Autodesk Inventor part; units mm, degrees
(part 2 of 3)
sketch "Sketch14" plane through (-2.25, 0, -155) normal (0, 0, -1) x (-1, 0, 0)
  line L0 (27.5213, 34.6376) -> (93.9787, 34.6376) construction
  line L1 (93.9787, 34.6376) -> (93.9787, 30.375) construction
  line L2 (93.9787, 30.375) -> (27.5213, 30.375) construction
  line L3 (27.5213, 30.375) -> (27.5213, 34.6376) construction
  line L4 (107.75, 0) -> (107.75, 55) projected
  circle A0 centre (60.75, 23) radius 5.375 projected
  spline S0 degree 2 poles (33.5458, 31.2786) (33.5458, 30.8312) (33.2054, 30.1457) (32.9234, 29.922) knots 0 0 0 1 2 2 2
  spline S1 degree 2 poles (32.9234, 29.922) (32.5831, 29.6594) (31.81, 29.4358) (31.1973, 29.4358) knots 0 0 0 1 2 2 2
  line L5 (31.1973, 29.4358) -> (29.4761, 29.4358)
  line L6 (29.4761, 29.4358) -> (29.4761, 35.4358)
  line L7 (29.4761, 35.4358) -> (31.066, 35.4358)
  spline S2 degree 2 poles (31.066, 35.4358) (31.7079, 35.4358) (32.3497, 35.3531) (32.6414, 35.1927) knots 0 0 0 1 2 2 2
  spline S3 degree 2 poles (32.6414, 35.1927) (32.9672, 35.0225) (33.2638, 34.4633) (33.2638, 34.0841) knots 0 0 0 1 2 2 2
  spline S4 degree 2 poles (33.2638, 34.0841) (33.2638, 33.6611) (32.8164, 32.9901) (32.4226, 32.8004) knots 0 0 0 1 2 2 2
  line L8 (32.4226, 32.8004) -> (32.4226, 32.7713)
  spline S5 degree 2 poles (32.4226, 32.7713) (32.9575, 32.6254) (33.5458, 31.8523) (33.5458, 31.2786) knots 0 0 0 1 2 2 2
  spline S6 degree 2 poles (32.7143, 31.2445) (32.7143, 31.5849) (32.5199, 32.0225) (32.2281, 32.1781) knots 0 0 0 1 2 2 2
  spline S7 degree 2 poles (32.2281, 32.1781) (32.0385, 32.2753) (31.5912, 32.3337) (31.1779, 32.3337) knots 0 0 0 1 2 2 2
  line L9 (31.1779, 32.3337) -> (30.2735, 32.3337)
  line L10 (30.2735, 32.3337) -> (30.2735, 30.1165)
  line L11 (30.2735, 30.1165) -> (30.9202, 30.1165)
  spline S8 degree 2 poles (30.9202, 30.1165) (31.4453, 30.1165) (32.0482, 30.2137) (32.2816, 30.3693) knots 0 0 0 1 2 2 2
  spline S9 degree 2 poles (32.2816, 30.3693) (32.5053, 30.5298) (32.7143, 30.9285) (32.7143, 31.2445) knots 0 0 0 1 2 2 2
  spline S10 degree 2 poles (32.4323, 33.9722) (32.4323, 34.1862) (32.2865, 34.5071) (32.126, 34.5995) knots 0 0 0 1 2 2 2
  spline S11 degree 2 poles (32.126, 34.5995) (31.9315, 34.7064) (31.4599, 34.7551) (31.0369, 34.7551) knots 0 0 0 1 2 2 2
  line L12 (31.0369, 34.7551) -> (30.2735, 34.7551)
  line L13 (30.2735, 34.7551) -> (30.2735, 32.9998)
  line L14 (30.2735, 32.9998) -> (31.1779, 32.9998)
  spline S12 degree 2 poles (31.1779, 32.9998) (31.5523, 32.9998) (31.9072, 33.0776) (32.0968, 33.1991) knots 0 0 0 1 2 2 2
  spline S13 degree 2 poles (32.0968, 33.1991) (32.2816, 33.3158) (32.4323, 33.6902) (32.4323, 33.9722) knots 0 0 0 1 2 2 2
  spline S14 degree 2 poles (36.7889, 29.9123) (36.6965, 29.8442) (36.3853, 29.6011) (36.2395, 29.5282) knots 0 0 0 1 2 2 2
  spline S15 degree 2 poles (36.2395, 29.5282) (36.0401, 29.4212) (35.6657, 29.3094) (35.3254, 29.3094) knots 0 0 0 1 2 2 2
  spline S16 degree 2 poles (35.3254, 29.3094) (35.0482, 29.3094) (34.5474, 29.5184) (34.3578, 29.7081) knots 0 0 0 1 2 2 2
  spline S17 degree 2 poles (34.3578, 29.7081) (34.1779, 29.8928) (33.9591, 30.4374) (33.9591, 30.7389) knots 0 0 0 1 2 2 2
  spline S18 degree 2 poles (33.9591, 30.7389) (33.9591, 31.2056) (34.3529, 31.8669) (34.7808, 32.0565) knots 0 0 0 1 2 2 2
  spline S19 degree 2 poles (34.7808, 32.0565) (35.16, 32.2316) (36.1908, 32.3628) (36.7889, 32.3969) knots 0 0 0 1 2 2 2
  line L15 (36.7889, 32.3969) -> (36.7889, 32.5427)
  spline S20 degree 2 poles (36.7889, 32.5427) (36.7889, 32.8053) (36.6284, 33.1311) (36.4826, 33.2235) knots 0 0 0 1 2 2 2
  spline S21 degree 2 poles (36.4826, 33.2235) (36.3367, 33.3158) (35.9186, 33.3742) (35.6949, 33.3742) knots 0 0 0 1 2 2 2
  spline S22 degree 2 poles (35.6949, 33.3742) (35.4323, 33.3742) (34.7224, 33.2186) (34.3675, 33.0679) knots 0 0 0 1 2 2 2
  line L16 (34.3675, 33.0679) -> (34.3237, 33.0679)
  line L17 (34.3237, 33.0679) -> (34.3237, 33.841)
  spline S23 degree 2 poles (34.3237, 33.841) (34.5328, 33.8993) (35.3156, 34.0452) (35.6998, 34.0452) knots 0 0 0 1 2 2 2
  spline S24 degree 2 poles (35.6998, 34.0452) (36.1665, 34.0452) (36.8035, 33.8993) (37.0563, 33.7097) knots 0 0 0 1 2 2 2
  spline S25 degree 2 poles (37.0563, 33.7097) (37.3043, 33.5249) (37.5474, 32.9366) (37.5474, 32.5136) knots 0 0 0 1 2 2 2
  line L18 (37.5474, 32.5136) -> (37.5474, 29.4358)
  line L19 (37.5474, 29.4358) -> (36.7889, 29.4358)
  line L20 (36.7889, 29.4358) -> (36.7889, 29.9123)
  line L21 (36.7889, 30.5444) -> (36.7889, 31.794)
  spline S26 degree 2 poles (36.7889, 31.794) (36.5166, 31.7697) (35.6949, 31.687) (35.4372, 31.6092) knots 0 0 0 1 2 2 2
  spline S27 degree 2 poles (35.4372, 31.6092) (35.1357, 31.5168) (34.7419, 31.1327) (34.7419, 30.7923) knots 0 0 0 1 2 2 2
  spline S28 degree 2 poles (34.7419, 30.7923) (34.7419, 30.4034) (35.1795, 30.0095) (35.5976, 30.0095) knots 0 0 0 1 2 2 2
  spline S29 degree 2 poles (35.5976, 30.0095) (35.9526, 30.0095) (36.5361, 30.3158) (36.7889, 30.5444) knots 0 0 0 1 2 2 2
  line L22 (40.9996, 33.1262) -> (40.9607, 33.1262)
  spline S30 degree 2 poles (40.9607, 33.1262) (40.8732, 33.1505) (40.6835, 33.1603) (40.5523, 33.1603) knots 0 0 0 1 2 2 2
  spline S31 degree 2 poles (40.5523, 33.1603) (40.2459, 33.1603) (39.643, 32.8928) (39.3707, 32.6303) knots 0 0 0 1 2 2 2
  line L23 (39.3707, 32.6303) -> (39.3707, 29.4358)
  line L24 (39.3707, 29.4358) -> (38.6122, 29.4358)
  line L25 (38.6122, 29.4358) -> (38.6122, 33.9382)
  line L26 (38.6122, 33.9382) -> (39.3707, 33.9382)
  line L27 (39.3707, 33.9382) -> (39.3707, 33.2672)
  spline S32 degree 2 poles (39.3707, 33.2672) (39.784, 33.6368) (40.4015, 33.9382) (40.6933, 33.9382) knots 0 0 0 1 2 2 2
  spline S33 degree 2 poles (40.6933, 33.9382) (40.81, 33.9382) (40.9267, 33.9285) (40.9996, 33.9139) knots 0 0 0 1 2 2 2
  line L28 (40.9996, 33.9139) -> (40.9996, 33.1262)
  line L29 (43.9753, 33.1262) -> (43.9364, 33.1262)
  spline S34 degree 2 poles (43.9364, 33.1262) (43.8489, 33.1505) (43.6592, 33.1603) (43.528, 33.1603) knots 0 0 0 1 2 2 2
  spline S35 degree 2 poles (43.528, 33.1603) (43.2216, 33.1603) (42.6187, 32.8928) (42.3464, 32.6303) knots 0 0 0 1 2 2 2
  line L30 (42.3464, 32.6303) -> (42.3464, 29.4358)
  line L31 (42.3464, 29.4358) -> (41.5879, 29.4358)
  line L32 (41.5879, 29.4358) -> (41.5879, 33.9382)
  line L33 (41.5879, 33.9382) -> (42.3464, 33.9382)
  line L34 (42.3464, 33.9382) -> (42.3464, 33.2672)
  spline S36 degree 2 poles (42.3464, 33.2672) (42.7597, 33.6368) (43.3772, 33.9382) (43.669, 33.9382) knots 0 0 0 1 2 2 2
  spline S37 degree 2 poles (43.669, 33.9382) (43.7857, 33.9382) (43.9023, 33.9285) (43.9753, 33.9139) knots 0 0 0 1 2 2 2
  line L35 (43.9753, 33.9139) -> (43.9753, 33.1262)
  spline S38 degree 2 poles (46.5182, 29.3337) (45.4388, 29.3337) (44.2524, 30.5444) (44.2524, 31.6627) knots 0 0 0 1 2 2 2
  spline S39 degree 2 poles (44.2524, 31.6627) (44.2524, 32.7615) (45.4048, 34.0646) (46.3335, 34.0646) knots 0 0 0 1 2 2 2
  spline S40 degree 2 poles (46.3335, 34.0646) (46.7516, 34.0646) (47.3983, 33.8215) (47.6365, 33.5638) knots 0 0 0 1 2 2 2
  spline S41 degree 2 poles (47.6365, 33.5638) (47.8797, 33.3061) (48.1374, 32.5622) (48.1374, 32.0225) knots 0 0 0 1 2 2 2
  line L36 (48.1374, 32.0225) -> (48.1374, 31.6092)
  line L37 (48.1374, 31.6092) -> (45.0207, 31.6092)
  spline S42 degree 2 poles (45.0207, 31.6092) (45.0207, 30.8264) (45.8083, 29.9949) (46.5085, 29.9949) knots 0 0 0 1 2 2 2
  spline S43 degree 2 poles (46.5085, 29.9949) (46.7565, 29.9949) (47.2378, 30.1068) (47.4323, 30.1943) knots 0 0 0 1 2 2 2
  spline S44 degree 2 poles (47.4323, 30.1943) (47.6365, 30.2915) (47.9186, 30.4617) (48.0109, 30.5395) knots 0 0 0 1 2 2 2
  line L38 (48.0109, 30.5395) -> (48.0547, 30.5395)
  line L39 (48.0547, 30.5395) -> (48.0547, 29.7129)
  spline S45 degree 2 poles (48.0547, 29.7129) (47.9234, 29.6594) (47.5247, 29.5038) (47.3691, 29.4601) knots 0 0 0 1 2 2 2
  spline S46 degree 2 poles (47.3691, 29.4601) (47.1503, 29.3969) (46.7905, 29.3337) (46.5182, 29.3337) knots 0 0 0 1 2 2 2
  spline S47 degree 2 poles (47.3983, 32.1878) (47.3886, 32.4941) (47.2622, 32.9415) (47.1406, 33.0922) knots 0 0 0 1 2 2 2
  spline S48 degree 2 poles (47.1406, 33.0922) (47.0093, 33.2624) (46.596, 33.4423) (46.2897, 33.4423) knots 0 0 0 1 2 2 2
  spline S49 degree 2 poles (46.2897, 33.4423) (45.9882, 33.4423) (45.5652, 33.2624) (45.3902, 33.0873) knots 0 0 0 1 2 2 2
  spline S50 degree 2 poles (45.3902, 33.0873) (45.22, 32.9074) (45.045, 32.4747) (45.0207, 32.1878) knots 0 0 0 1 2 2 2
  line L40 (45.0207, 32.1878) -> (47.3983, 32.1878)
  line L41 (49.6787, 29.4358) -> (48.9202, 29.4358)
  line L42 (48.9202, 29.4358) -> (48.9202, 35.7032)
  line L43 (48.9202, 35.7032) -> (49.6787, 35.7032)
  line L44 (49.6787, 35.7032) -> (49.6787, 29.4358)
  spline S51 degree 2 poles (57.22, 33.627) (57.22, 33.238) (56.9429, 32.5379) (56.6949, 32.2948) knots 0 0 0 1 2 2 2
  spline S52 degree 2 poles (56.6949, 32.2948) (56.3837, 31.9885) (55.5425, 31.6724) (54.9007, 31.6724) knots 0 0 0 1 2 2 2
  line L45 (54.9007, 31.6724) -> (54.2249, 31.6724)
  line L46 (54.2249, 31.6724) -> (54.2249, 29.4358)
  line L47 (54.2249, 29.4358) -> (53.4275, 29.4358)
  line L48 (53.4275, 29.4358) -> (53.4275, 35.4358)
  line L49 (53.4275, 35.4358) -> (54.9348, 35.4358)
  spline S53 degree 2 poles (54.9348, 35.4358) (55.4696, 35.4358) (56.2184, 35.2607) (56.5053, 35.0614) knots 0 0 0 1 2 2 2
  spline S54 degree 2 poles (56.5053, 35.0614) (56.8408, 34.8329) (57.22, 34.1278) (57.22, 33.627) knots 0 0 0 1 2 2 2
  spline S55 degree 2 poles (56.3886, 33.6027) (56.3886, 33.9139) (56.1746, 34.3709) (55.9558, 34.5168) knots 0 0 0 1 2 2 2
  spline S56 degree 2 poles (55.9558, 34.5168) (55.7662, 34.6432) (55.2605, 34.7453) (54.8861, 34.7453) knots 0 0 0 1 2 2 2
  line L50 (54.8861, 34.7453) -> (54.2249, 34.7453)
  line L51 (54.2249, 34.7453) -> (54.2249, 32.3531)
  line L52 (54.2249, 32.3531) -> (54.7694, 32.3531)
  spline S57 degree 2 poles (54.7694, 32.3531) (55.2557, 32.3531) (55.8537, 32.5087) (56.0482, 32.7129) knots 0 0 0 1 2 2 2
  spline S58 degree 2 poles (56.0482, 32.7129) (56.2281, 32.8928) (56.3886, 33.3158) (56.3886, 33.6027) knots 0 0 0 1 2 2 2
  spline S59 degree 2 poles (61.6203, 31.687) (61.6203, 30.5492) (60.5263, 29.3094) (59.6122, 29.3094) knots 0 0 0 1 2 2 2
  spline S60 degree 2 poles (59.6122, 29.3094) (58.6738, 29.3094) (57.5993, 30.5881) (57.5993, 31.687) knots 0 0 0 1 2 2 2
  spline S61 degree 2 poles (57.5993, 31.687) (57.5993, 32.815) (58.7079, 34.0646) (59.6122, 34.0646) knots 0 0 0 1 2 2 2
  spline S62 degree 2 poles (59.6122, 34.0646) (60.5263, 34.0646) (61.6203, 32.8199) (61.6203, 31.687) knots 0 0 0 1 2 2 2
  spline S63 degree 2 poles (60.8375, 31.687) (60.8375, 32.5622) (60.2006, 33.4131) (59.6122, 33.4131) knots 0 0 0 1 2 2 2
  spline S64 degree 2 poles (59.6122, 33.4131) (59.0239, 33.4131) (58.3821, 32.5622) (58.3821, 31.687) knots 0 0 0 1 2 2 2
  spline S65 degree 2 poles (58.3821, 31.687) (58.3821, 30.8361) (59.0239, 29.9609) (59.6122, 29.9609) knots 0 0 0 1 2 2 2
  spline S66 degree 2 poles (59.6122, 29.9609) (60.1957, 29.9609) (60.8375, 30.8215) (60.8375, 31.687) knots 0 0 0 1 2 2 2
  line L53 (67.8537, 33.9382) -> (66.7111, 29.4358)
  line L54 (66.7111, 29.4358) -> (66.0109, 29.4358)
  line L55 (66.0109, 29.4358) -> (64.9121, 32.9074)
  line L56 (64.9121, 32.9074) -> (63.8181, 29.4358)
  line L57 (63.8181, 29.4358) -> (63.1228, 29.4358)
  line L58 (63.1228, 29.4358) -> (61.9704, 33.9382)
  line L59 (61.9704, 33.9382) -> (62.7581, 33.9382)
  line L60 (62.7581, 33.9382) -> (63.5555, 30.452)
  line L61 (63.5555, 30.452) -> (64.6203, 33.9382)
  line L62 (64.6203, 33.9382) -> (65.2476, 33.9382)
  line L63 (65.2476, 33.9382) -> (66.3416, 30.452)
  line L64 (66.3416, 30.452) -> (67.0904, 33.9382)
  line L65 (67.0904, 33.9382) -> (67.8537, 33.9382)
  spline S67 degree 2 poles (70.4745, 29.3337) (69.3951, 29.3337) (68.2087, 30.5444) (68.2087, 31.6627) knots 0 0 0 1 2 2 2
  spline S68 degree 2 poles (68.2087, 31.6627) (68.2087, 32.7615) (69.361, 34.0646) (70.2897, 34.0646) knots 0 0 0 1 2 2 2
  spline S69 degree 2 poles (70.2897, 34.0646) (70.7079, 34.0646) (71.3545, 33.8215) (71.5928, 33.5638) knots 0 0 0 1 2 2 2
  spline S70 degree 2 poles (71.5928, 33.5638) (71.8359, 33.3061) (72.0936, 32.5622) (72.0936, 32.0225) knots 0 0 0 1 2 2 2
  line L66 (72.0936, 32.0225) -> (72.0936, 31.6092)
  line L67 (72.0936, 31.6092) -> (68.9769, 31.6092)
  spline S71 degree 2 poles (68.9769, 31.6092) (68.9769, 30.8264) (69.7646, 29.9949) (70.4647, 29.9949) knots 0 0 0 1 2 2 2
  spline S72 degree 2 poles (70.4647, 29.9949) (70.7127, 29.9949) (71.1941, 30.1068) (71.3886, 30.1943) knots 0 0 0 1 2 2 2
  spline S73 degree 2 poles (71.3886, 30.1943) (71.5928, 30.2915) (71.8748, 30.4617) (71.9672, 30.5395) knots 0 0 0 1 2 2 2
  line L68 (71.9672, 30.5395) -> (72.0109, 30.5395)
  line L69 (72.0109, 30.5395) -> (72.0109, 29.7129)
  spline S74 degree 2 poles (72.0109, 29.7129) (71.8797, 29.6594) (71.481, 29.5038) (71.3254, 29.4601) knots 0 0 0 1 2 2 2
  spline S75 degree 2 poles (71.3254, 29.4601) (71.1066, 29.3969) (70.7468, 29.3337) (70.4745, 29.3337) knots 0 0 0 1 2 2 2
  spline S76 degree 2 poles (71.3545, 32.1878) (71.3448, 32.4941) (71.2184, 32.9415) (71.0968, 33.0922) knots 0 0 0 1 2 2 2
  spline S77 degree 2 poles (71.0968, 33.0922) (70.9656, 33.2624) (70.5523, 33.4423) (70.2459, 33.4423) knots 0 0 0 1 2 2 2
  spline S78 degree 2 poles (70.2459, 33.4423) (69.9445, 33.4423) (69.5215, 33.2624) (69.3464, 33.0873) knots 0 0 0 1 2 2 2
  spline S79 degree 2 poles (69.3464, 33.0873) (69.1763, 32.9074) (69.0012, 32.4747) (68.9769, 32.1878) knots 0 0 0 1 2 2 2
  line L70 (68.9769, 32.1878) -> (71.3545, 32.1878)
  line L71 (75.2492, 33.1262) -> (75.2103, 33.1262)
  spline S80 degree 2 poles (75.2103, 33.1262) (75.1228, 33.1505) (74.9331, 33.1603) (74.8019, 33.1603) knots 0 0 0 1 2 2 2
  spline S81 degree 2 poles (74.8019, 33.1603) (74.4955, 33.1603) (73.8926, 32.8928) (73.6203, 32.6303) knots 0 0 0 1 2 2 2
  line L72 (73.6203, 32.6303) -> (73.6203, 29.4358)
  line L73 (73.6203, 29.4358) -> (72.8618, 29.4358)
  line L74 (72.8618, 29.4358) -> (72.8618, 33.9382)
  line L75 (72.8618, 33.9382) -> (73.6203, 33.9382)
  line L76 (73.6203, 33.9382) -> (73.6203, 33.2672)
  spline S82 degree 2 poles (73.6203, 33.2672) (74.0336, 33.6368) (74.6511, 33.9382) (74.9429, 33.9382) knots 0 0 0 1 2 2 2
  spline S83 degree 2 poles (74.9429, 33.9382) (75.0596, 33.9382) (75.1763, 33.9285) (75.2492, 33.9139) knots 0 0 0 1 2 2 2
  line L77 (75.2492, 33.9139) -> (75.2492, 33.1262)
  spline S84 degree 2 poles (82.2654, 33.627) (82.2654, 33.238) (81.9882, 32.5379) (81.7403, 32.2948) knots 0 0 0 1 2 2 2
  spline S85 degree 2 poles (81.7403, 32.2948) (81.4291, 31.9885) (80.5879, 31.6724) (79.9461, 31.6724) knots 0 0 0 1 2 2 2
  line L78 (79.9461, 31.6724) -> (79.2703, 31.6724)
  line L79 (79.2703, 31.6724) -> (79.2703, 29.4358)
  line L80 (79.2703, 29.4358) -> (78.4729, 29.4358)
  line L81 (78.4729, 29.4358) -> (78.4729, 35.4358)
  line L82 (78.4729, 35.4358) -> (79.9801, 35.4358)
  spline S86 degree 2 poles (79.9801, 35.4358) (80.515, 35.4358) (81.2638, 35.2607) (81.5506, 35.0614) knots 0 0 0 1 2 2 2
  spline S87 degree 2 poles (81.5506, 35.0614) (81.8861, 34.8329) (82.2654, 34.1278) (82.2654, 33.627) knots 0 0 0 1 2 2 2
  spline S88 degree 2 poles (81.434, 33.6027) (81.434, 33.9139) (81.22, 34.3709) (81.0012, 34.5168) knots 0 0 0 1 2 2 2
  spline S89 degree 2 poles (81.0012, 34.5168) (80.8116, 34.6432) (80.3059, 34.7453) (79.9315, 34.7453) knots 0 0 0 1 2 2 2
  line L83 (79.9315, 34.7453) -> (79.2703, 34.7453)
  line L84 (79.2703, 34.7453) -> (79.2703, 32.3531)
  line L85 (79.2703, 32.3531) -> (79.8148, 32.3531)
  spline S90 degree 2 poles (79.8148, 32.3531) (80.3011, 32.3531) (80.8991, 32.5087) (81.0936, 32.7129) knots 0 0 0 1 2 2 2
  spline S91 degree 2 poles (81.0936, 32.7129) (81.2735, 32.8928) (81.434, 33.3158) (81.434, 33.6027) knots 0 0 0 1 2 2 2
  spline S92 degree 2 poles (86.6657, 31.687) (86.6657, 30.5492) (85.5717, 29.3094) (84.6576, 29.3094) knots 0 0 0 1 2 2 2
  spline S93 degree 2 poles (84.6576, 29.3094) (83.7192, 29.3094) (82.6447, 30.5881) (82.6447, 31.687) knots 0 0 0 1 2 2 2
  spline S94 degree 2 poles (82.6447, 31.687) (82.6447, 32.815) (83.7532, 34.0646) (84.6576, 34.0646) knots 0 0 0 1 2 2 2
  spline S95 degree 2 poles (84.6576, 34.0646) (85.5717, 34.0646) (86.6657, 32.8199) (86.6657, 31.687) knots 0 0 0 1 2 2 2
  spline S96 degree 2 poles (85.8829, 31.687) (85.8829, 32.5622) (85.2459, 33.4131) (84.6576, 33.4131) knots 0 0 0 1 2 2 2
  spline S97 degree 2 poles (84.6576, 33.4131) (84.0693, 33.4131) (83.4275, 32.5622) (83.4275, 31.687) knots 0 0 0 1 2 2 2
  spline S98 degree 2 poles (83.4275, 31.687) (83.4275, 30.8361) (84.0693, 29.9609) (84.6576, 29.9609) knots 0 0 0 1 2 2 2
  spline S99 degree 2 poles (84.6576, 29.9609) (85.2411, 29.9609) (85.8829, 30.8215) (85.8829, 31.687) knots 0 0 0 1 2 2 2
  line L86 (89.831, 33.1262) -> (89.7921, 33.1262)
  spline S100 degree 2 poles (89.7921, 33.1262) (89.7046, 33.1505) (89.515, 33.1603) (89.3837, 33.1603) knots 0 0 0 1 2 2 2
  spline S101 degree 2 poles (89.3837, 33.1603) (89.0774, 33.1603) (88.4745, 32.8928) (88.2022, 32.6303) knots 0 0 0 1 2 2 2
  line L87 (88.2022, 32.6303) -> (88.2022, 29.4358)
  line L88 (88.2022, 29.4358) -> (87.4437, 29.4358)
  line L89 (87.4437, 29.4358) -> (87.4437, 33.9382)
  line L90 (87.4437, 33.9382) -> (88.2022, 33.9382)
  line L91 (88.2022, 33.9382) -> (88.2022, 33.2672)
  spline S102 degree 2 poles (88.2022, 33.2672) (88.6155, 33.6368) (89.233, 33.9382) (89.5247, 33.9382) knots 0 0 0 1 2 2 2
  spline S103 degree 2 poles (89.5247, 33.9382) (89.6414, 33.9382) (89.7581, 33.9285) (89.831, 33.9139) knots 0 0 0 1 2 2 2
  line L92 (89.831, 33.9139) -> (89.831, 33.1262)
  spline S104 degree 2 poles (91.7808, 29.3483) (91.1633, 29.3483) (90.468, 30.0533) (90.468, 30.8167) knots 0 0 0 1 2 2 2
  line L93 (90.468, 30.8167) -> (90.468, 33.311)
  line L94 (90.468, 33.311) -> (89.9575, 33.311)
  line L95 (89.9575, 33.311) -> (89.9575, 33.9382)
  line L96 (89.9575, 33.9382) -> (90.468, 33.9382)
  line L97 (90.468, 33.9382) -> (90.468, 35.2316)
  line L98 (90.468, 35.2316) -> (91.2265, 35.2316)
  line L99 (91.2265, 35.2316) -> (91.2265, 33.9382)
  line L100 (91.2265, 33.9382) -> (92.622, 33.9382)
  line L101 (92.622, 33.9382) -> (92.622, 33.311)
  line L102 (92.622, 33.311) -> (91.2265, 33.311)
  line L103 (91.2265, 33.311) -> (91.2265, 31.1667)
  spline S105 degree 2 poles (91.2265, 31.1667) (91.2265, 30.8264) (91.2508, 30.452) (91.3335, 30.2915) knots 0 0 0 1 2 2 2
  spline S106 degree 2 poles (91.3335, 30.2915) (91.4015, 30.1505) (91.7079, 30.0095) (91.9704, 30.0095) knots 0 0 0 1 2 2 2
  spline S107 degree 2 poles (91.9704, 30.0095) (92.1552, 30.0095) (92.5004, 30.1214) (92.5782, 30.1554) knots 0 0 0 1 2 2 2
  line L104 (92.5782, 30.1554) -> (92.622, 30.1554)
  line L105 (92.622, 30.1554) -> (92.622, 29.4747)
  spline S108 degree 2 poles (92.622, 29.4747) (92.408, 29.4163) (91.9704, 29.3483) (91.7808, 29.3483) knots 0 0 0 1 2 2 2
  point P0 (-2.25, 0)
  point P1 (60.75, 30.375)
  dimension "d140" = 47
  dimension "d143" = 7.375
  constraints: 1 midpoint, 2 other
  measures "d140" distance from line of L4 point (60.75, 30.375)
  measures "d143" distance of A0.centre point (60.75, 30.375)
sketch "Sketch15" plane through (-110, 0, -152.75) normal (-1, 0, 0) x (0, 0, 1)
  line L0 (69.7148, 46.767) -> (124.7852, 46.767) construction
  line L1 (124.7852, 46.767) -> (124.7852, 42.3) construction
  line L2 (124.7852, 42.3) -> (69.7148, 42.3) construction
  line L3 (69.7148, 42.3) -> (69.7148, 46.767) construction
  line L4 (90.75, 40.3) -> (103.75, 40.3) projected
  line L5 (75.8537, 41.5432) -> (75.0563, 41.5432)
  line L6 (75.0563, 41.5432) -> (75.0563, 46.7118)
  line L7 (75.0563, 46.7118) -> (73.4907, 43.1964)
  line L8 (73.4907, 43.1964) -> (73.0045, 43.1964)
  line L9 (73.0045, 43.1964) -> (71.4534, 46.7118)
  line L10 (71.4534, 46.7118) -> (71.4534, 41.5432)
  line L11 (71.4534, 41.5432) -> (70.7095, 41.5432)
  line L12 (70.7095, 41.5432) -> (70.7095, 47.5432)
  line L13 (70.7095, 47.5432) -> (71.7986, 47.5432)
  line L14 (71.7986, 47.5432) -> (73.2962, 44.2029)
  line L15 (73.2962, 44.2029) -> (74.7451, 47.5432)
  line L16 (74.7451, 47.5432) -> (75.8537, 47.5432)
  line L17 (75.8537, 47.5432) -> (75.8537, 41.5432)
  line L18 (77.784, 41.5432) -> (77.0255, 41.5432)
  line L19 (77.0255, 41.5432) -> (77.0255, 46.0457)
  line L20 (77.0255, 46.0457) -> (77.784, 46.0457)
  line L21 (77.784, 46.0457) -> (77.784, 41.5432)
  line L22 (77.8375, 46.7944) -> (76.9769, 46.7944)
  line L23 (76.9769, 46.7944) -> (76.9769, 47.5821)
  line L24 (76.9769, 47.5821) -> (77.8375, 47.5821)
  line L25 (77.8375, 47.5821) -> (77.8375, 46.7944)
  line L26 (81.2848, 45.2337) -> (81.2459, 45.2337)
  spline S0 degree 2 poles (81.2459, 45.2337) (81.1584, 45.258) (80.9688, 45.2677) (80.8375, 45.2677) knots 0 0 0 1 2 2 2
  spline S1 degree 2 poles (80.8375, 45.2677) (80.5312, 45.2677) (79.9283, 45.0003) (79.656, 44.7377) knots 0 0 0 1 2 2 2
  line L27 (79.656, 44.7377) -> (79.656, 41.5432)
  line L28 (79.656, 41.5432) -> (78.8975, 41.5432)
  line L29 (78.8975, 41.5432) -> (78.8975, 46.0457)
  line L30 (78.8975, 46.0457) -> (79.656, 46.0457)
  line L31 (79.656, 46.0457) -> (79.656, 45.3747)
  spline S2 degree 2 poles (79.656, 45.3747) (80.0693, 45.7442) (80.6868, 46.0457) (80.9785, 46.0457) knots 0 0 0 1 2 2 2
  spline S3 degree 2 poles (80.9785, 46.0457) (81.0952, 46.0457) (81.2119, 46.0359) (81.2848, 46.0213) knots 0 0 0 1 2 2 2
  line L32 (81.2848, 46.0213) -> (81.2848, 45.2337)
  spline S4 degree 2 poles (83.6625, 41.4411) (83.1957, 41.4411) (82.4226, 41.728) (82.1455, 42.0197) knots 0 0 0 1 2 2 2
  spline S5 degree 2 poles (82.1455, 42.0197) (81.8683, 42.3066) (81.562, 43.1915) (81.562, 43.7847) knots 0 0 0 1 2 2 2
  spline S6 degree 2 poles (81.562, 43.7847) (81.562, 44.3779) (81.878, 45.2434) (82.1455, 45.5351) knots 0 0 0 1 2 2 2
  spline S7 degree 2 poles (82.1455, 45.5351) (82.4129, 45.8317) (83.2054, 46.1478) (83.6625, 46.1478) knots 0 0 0 1 2 2 2
  spline S8 degree 2 poles (83.6625, 46.1478) (84.032, 46.1478) (84.7224, 45.9387) (84.9899, 45.8025) knots 0 0 0 1 2 2 2
  line L33 (84.9899, 45.8025) -> (84.9899, 44.9517)
  line L34 (84.9899, 44.9517) -> (84.9461, 44.9517)
  spline S9 degree 2 poles (84.9461, 44.9517) (84.8635, 45.0197) (84.6106, 45.1948) (84.4307, 45.2871) knots 0 0 0 1 2 2 2
  spline S10 degree 2 poles (84.4307, 45.2871) (84.2703, 45.3649) (83.8424, 45.4865) (83.6479, 45.4865) knots 0 0 0 1 2 2 2
  spline S11 degree 2 poles (83.6479, 45.4865) (83.0596, 45.4865) (82.3448, 44.5967) (82.3448, 43.7847) knots 0 0 0 1 2 2 2
  spline S12 degree 2 poles (82.3448, 43.7847) (82.3448, 42.9922) (83.0353, 42.1024) (83.6479, 42.1024) knots 0 0 0 1 2 2 2
  spline S13 degree 2 poles (83.6479, 42.1024) (84.0174, 42.1024) (84.6884, 42.4087) (84.9461, 42.647) knots 0 0 0 1 2 2 2
  line L35 (84.9461, 42.647) -> (84.9899, 42.647)
  line L36 (84.9899, 42.647) -> (84.9899, 41.7961)
  spline S14 degree 2 poles (84.9899, 41.7961) (84.878, 41.7426) (84.5377, 41.5918) (84.4015, 41.5578) knots 0 0 0 1 2 2 2
  spline S15 degree 2 poles (84.4015, 41.5578) (84.207, 41.4995) (83.9007, 41.4411) (83.6625, 41.4411) knots 0 0 0 1 2 2 2
  spline S16 degree 2 poles (89.3805, 43.7944) (89.3805, 42.6567) (88.2865, 41.4168) (87.3724, 41.4168) knots 0 0 0 1 2 2 2
  spline S17 degree 2 poles (87.3724, 41.4168) (86.434, 41.4168) (85.3594, 42.6956) (85.3594, 43.7944) knots 0 0 0 1 2 2 2
  spline S18 degree 2 poles (85.3594, 43.7944) (85.3594, 44.9225) (86.468, 46.1721) (87.3724, 46.1721) knots 0 0 0 1 2 2 2
  spline S19 degree 2 poles (87.3724, 46.1721) (88.2865, 46.1721) (89.3805, 44.9273) (89.3805, 43.7944) knots 0 0 0 1 2 2 2
  spline S20 degree 2 poles (88.5976, 43.7944) (88.5976, 44.6696) (87.9607, 45.5205) (87.3724, 45.5205) knots 0 0 0 1 2 2 2
  spline S21 degree 2 poles (87.3724, 45.5205) (86.784, 45.5205) (86.1422, 44.6696) (86.1422, 43.7944) knots 0 0 0 1 2 2 2
  spline S22 degree 2 poles (86.1422, 43.7944) (86.1422, 42.9435) (86.784, 42.0683) (87.3724, 42.0683) knots 0 0 0 1 2 2 2
  spline S23 degree 2 poles (87.3724, 42.0683) (87.9558, 42.0683) (88.5976, 42.929) (88.5976, 43.7944) knots 0 0 0 1 2 2 2
  spline S24 degree 2 poles (94.8894, 41.4168) (94.3594, 41.4168) (93.5717, 41.694) (93.2946, 41.9711) knots 0 0 0 1 2 2 2
  spline S25 degree 2 poles (93.2946, 41.9711) (92.9785, 42.2823) (92.7208, 43.1575) (92.7208, 43.7993) knots 0 0 0 1 2 2 2
  line L37 (92.7208, 43.7993) -> (92.7208, 47.5432)
  line L38 (92.7208, 47.5432) -> (93.5182, 47.5432)
  line L39 (93.5182, 47.5432) -> (93.5182, 43.7993)
  spline S26 degree 2 poles (93.5182, 43.7993) (93.5182, 43.3812) (93.6252, 42.8171) (93.7759, 42.5886) knots 0 0 0 1 2 2 2
  spline S27 degree 2 poles (93.7759, 42.5886) (93.9364, 42.3455) (94.4907, 42.0975) (94.8894, 42.0975) knots 0 0 0 1 2 2 2
  spline S28 degree 2 poles (94.8894, 42.0975) (95.2638, 42.0975) (95.8472, 42.3455) (96.0077, 42.5886) knots 0 0 0 1 2 2 2
  spline S29 degree 2 poles (96.0077, 42.5886) (96.1584, 42.8171) (96.2654, 43.3763) (96.2654, 43.7799) knots 0 0 0 1 2 2 2
  line L40 (96.2654, 43.7799) -> (96.2654, 47.5432)
  line L41 (96.2654, 47.5432) -> (97.0628, 47.5432)
  line L42 (97.0628, 47.5432) -> (97.0628, 43.7993)
  spline S30 degree 2 poles (97.0628, 43.7993) (97.0628, 43.1721) (96.81, 42.2774) (96.4891, 41.9711) knots 0 0 0 1 2 2 2
  spline S31 degree 2 poles (96.4891, 41.9711) (96.2022, 41.6891) (95.4437, 41.4168) (94.8894, 41.4168) knots 0 0 0 1 2 2 2
  spline S32 degree 2 poles (99.878, 41.4363) (99.2265, 41.4363) (98.3124, 41.7085) (97.9088, 41.903) knots 0 0 0 1 2 2 2
  line L43 (97.9088, 41.903) -> (97.9088, 42.9047)
  line L44 (97.9088, 42.9047) -> (97.9672, 42.9047)
  spline S33 degree 2 poles (97.9672, 42.9047) (98.361, 42.5351) (99.3578, 42.1267) (99.8197, 42.1267) knots 0 0 0 1 2 2 2
  spline S34 degree 2 poles (99.8197, 42.1267) (100.481, 42.1267) (101.1568, 42.6761) (101.1568, 43.1283) knots 0 0 0 1 2 2 2
  spline S35 degree 2 poles (101.1568, 43.1283) (101.1568, 43.4881) (100.8019, 43.9354) (100.4177, 44.0473) knots 0 0 0 1 2 2 2
  spline S36 degree 2 poles (100.4177, 44.0473) (100.1406, 44.1251) (99.6787, 44.232) (99.3335, 44.3196) knots 0 0 0 1 2 2 2
  spline S37 degree 2 poles (99.3335, 44.3196) (99.0223, 44.4022) (98.5312, 44.6502) (98.3416, 44.8495) knots 0 0 0 1 2 2 2
  spline S38 degree 2 poles (98.3416, 44.8495) (98.1568, 45.0489) (97.9526, 45.5837) (97.9526, 45.9338) knots 0 0 0 1 2 2 2
  spline S39 degree 2 poles (97.9526, 45.9338) (97.9526, 46.6632) (99.0904, 47.6502) (99.9704, 47.6502) knots 0 0 0 1 2 2 2
  spline S40 degree 2 poles (99.9704, 47.6502) (100.4761, 47.6502) (101.3707, 47.4508) (101.7549, 47.2612) knots 0 0 0 1 2 2 2
  line L45 (101.7549, 47.2612) -> (101.7549, 46.3082)
  line L46 (101.7549, 46.3082) -> (101.6965, 46.3082)
  spline S41 degree 2 poles (101.6965, 46.3082) (101.4096, 46.5708) (100.515, 46.9598) (100.0239, 46.9598) knots 0 0 0 1 2 2 2
  spline S42 degree 2 poles (100.0239, 46.9598) (99.4696, 46.9598) (98.784, 46.4395) (98.784, 46.0165) knots 0 0 0 1 2 2 2
  spline S43 degree 2 poles (98.784, 46.0165) (98.784, 45.6372) (99.1876, 45.185) (99.5669, 45.0829) knots 0 0 0 1 2 2 2
  spline S44 degree 2 poles (99.5669, 45.0829) (99.8197, 45.0149) (100.5539, 44.8398) (100.797, 44.7669) knots 0 0 0 1 2 2 2
  spline S45 degree 2 poles (100.797, 44.7669) (101.4145, 44.5773) (101.9882, 43.8139) (101.9882, 43.2547) knots 0 0 0 1 2 2 2
  spline S46 degree 2 poles (101.9882, 43.2547) (101.9882, 42.8998) (101.7014, 42.2191) (101.4437, 41.9808) knots 0 0 0 1 2 2 2
  spline S47 degree 2 poles (101.4437, 41.9808) (101.1568, 41.7183) (100.4275, 41.4363) (99.878, 41.4363) knots 0 0 0 1 2 2 2
  spline S48 degree 2 poles (106.8699, 43.386) (106.8699, 42.9387) (106.5296, 42.2531) (106.2476, 42.0294) knots 0 0 0 1 2 2 2
  spline S49 degree 2 poles (106.2476, 42.0294) (105.9072, 41.7669) (105.1341, 41.5432) (104.5215, 41.5432) knots 0 0 0 1 2 2 2
  line L47 (104.5215, 41.5432) -> (102.8002, 41.5432)
  line L48 (102.8002, 41.5432) -> (102.8002, 47.5432)
  line L49 (102.8002, 47.5432) -> (104.3902, 47.5432)
  spline S50 degree 2 poles (104.3902, 47.5432) (105.032, 47.5432) (105.6738, 47.4606) (105.9656, 47.3001) knots 0 0 0 1 2 2 2
  spline S51 degree 2 poles (105.9656, 47.3001) (106.2913, 47.1299) (106.5879, 46.5708) (106.5879, 46.1915) knots 0 0 0 1 2 2 2
  spline S52 degree 2 poles (106.5879, 46.1915) (106.5879, 45.7685) (106.1406, 45.0975) (105.7468, 44.9079) knots 0 0 0 1 2 2 2
  line L50 (105.7468, 44.9079) -> (105.7468, 44.8787)
  spline S53 degree 2 poles (105.7468, 44.8787) (106.2816, 44.7329) (106.8699, 43.9598) (106.8699, 43.386) knots 0 0 0 1 2 2 2
  spline S54 degree 2 poles (106.0385, 43.352) (106.0385, 43.6923) (105.844, 44.1299) (105.5523, 44.2855) knots 0 0 0 1 2 2 2
  spline S55 degree 2 poles (105.5523, 44.2855) (105.3626, 44.3828) (104.9153, 44.4411) (104.502, 44.4411) knots 0 0 0 1 2 2 2
  line L51 (104.502, 44.4411) -> (103.5977, 44.4411)
  line L52 (103.5977, 44.4411) -> (103.5977, 42.2239)
  line L53 (103.5977, 42.2239) -> (104.2443, 42.2239)
  spline S56 degree 2 poles (104.2443, 42.2239) (104.7694, 42.2239) (105.3724, 42.3212) (105.6058, 42.4768) knots 0 0 0 1 2 2 2
  spline S57 degree 2 poles (105.6058, 42.4768) (105.8294, 42.6372) (106.0385, 43.0359) (106.0385, 43.352) knots 0 0 0 1 2 2 2
  spline S58 degree 2 poles (105.7565, 46.0797) (105.7565, 46.2936) (105.6106, 46.6145) (105.4502, 46.7069) knots 0 0 0 1 2 2 2
  spline S59 degree 2 poles (105.4502, 46.7069) (105.2557, 46.8139) (104.784, 46.8625) (104.361, 46.8625) knots 0 0 0 1 2 2 2
  line L54 (104.361, 46.8625) -> (103.5977, 46.8625)
  line L55 (103.5977, 46.8625) -> (103.5977, 45.1072)
  line L56 (103.5977, 45.1072) -> (104.502, 45.1072)
  spline S60 degree 2 poles (104.502, 45.1072) (104.8764, 45.1072) (105.2314, 45.185) (105.421, 45.3066) knots 0 0 0 1 2 2 2
  spline S61 degree 2 poles (105.421, 45.3066) (105.6058, 45.4233) (105.7565, 45.7977) (105.7565, 46.0797) knots 0 0 0 1 2 2 2
  spline S62 degree 2 poles (114.032, 45.7345) (114.032, 45.3455) (113.7549, 44.6453) (113.5069, 44.4022) knots 0 0 0 1 2 2 2
  spline S63 degree 2 poles (113.5069, 44.4022) (113.1957, 44.0959) (112.3545, 43.7799) (111.7127, 43.7799) knots 0 0 0 1 2 2 2
  line L57 (111.7127, 43.7799) -> (111.0369, 43.7799)
  line L58 (111.0369, 43.7799) -> (111.0369, 41.5432)
  line L59 (111.0369, 41.5432) -> (110.2395, 41.5432)
  line L60 (110.2395, 41.5432) -> (110.2395, 47.5432)
  line L61 (110.2395, 47.5432) -> (111.7468, 47.5432)
  spline S64 degree 2 poles (111.7468, 47.5432) (112.2816, 47.5432) (113.0304, 47.3682) (113.3173, 47.1688) knots 0 0 0 1 2 2 2
  spline S65 degree 2 poles (113.3173, 47.1688) (113.6528, 46.9403) (114.032, 46.2353) (114.032, 45.7345) knots 0 0 0 1 2 2 2
  spline S66 degree 2 poles (113.2006, 45.7102) (113.2006, 46.0213) (112.9866, 46.4784) (112.7678, 46.6243) knots 0 0 0 1 2 2 2
  spline S67 degree 2 poles (112.7678, 46.6243) (112.5782, 46.7507) (112.0725, 46.8528) (111.6981, 46.8528) knots 0 0 0 1 2 2 2
  line L62 (111.6981, 46.8528) -> (111.0369, 46.8528)
  line L63 (111.0369, 46.8528) -> (111.0369, 44.4606)
  line L64 (111.0369, 44.4606) -> (111.5814, 44.4606)
  spline S68 degree 2 poles (111.5814, 44.4606) (112.0677, 44.4606) (112.6657, 44.6162) (112.8602, 44.8204) knots 0 0 0 1 2 2 2
  spline S69 degree 2 poles (112.8602, 44.8204) (113.0401, 45.0003) (113.2006, 45.4233) (113.2006, 45.7102) knots 0 0 0 1 2 2 2
  spline S70 degree 2 poles (118.4323, 43.7944) (118.4323, 42.6567) (117.3383, 41.4168) (116.4242, 41.4168) knots 0 0 0 1 2 2 2
  spline S71 degree 2 poles (116.4242, 41.4168) (115.4858, 41.4168) (114.4113, 42.6956) (114.4113, 43.7944) knots 0 0 0 1 2 2 2
  spline S72 degree 2 poles (114.4113, 43.7944) (114.4113, 44.9225) (115.5199, 46.1721) (116.4242, 46.1721) knots 0 0 0 1 2 2 2
  spline S73 degree 2 poles (116.4242, 46.1721) (117.3383, 46.1721) (118.4323, 44.9273) (118.4323, 43.7944) knots 0 0 0 1 2 2 2
  spline S74 degree 2 poles (117.6495, 43.7944) (117.6495, 44.6696) (117.0126, 45.5205) (116.4242, 45.5205) knots 0 0 0 1 2 2 2
  spline S75 degree 2 poles (116.4242, 45.5205) (115.8359, 45.5205) (115.1941, 44.6696) (115.1941, 43.7944) knots 0 0 0 1 2 2 2
  spline S76 degree 2 poles (115.1941, 43.7944) (115.1941, 42.9435) (115.8359, 42.0683) (116.4242, 42.0683) knots 0 0 0 1 2 2 2
  spline S77 degree 2 poles (116.4242, 42.0683) (117.0077, 42.0683) (117.6495, 42.929) (117.6495, 43.7944) knots 0 0 0 1 2 2 2
  line L65 (121.5977, 45.2337) -> (121.5588, 45.2337)
  spline S78 degree 2 poles (121.5588, 45.2337) (121.4712, 45.258) (121.2816, 45.2677) (121.1503, 45.2677) knots 0 0 0 1 2 2 2
  spline S79 degree 2 poles (121.1503, 45.2677) (120.844, 45.2677) (120.2411, 45.0003) (119.9688, 44.7377) knots 0 0 0 1 2 2 2
  line L66 (119.9688, 44.7377) -> (119.9688, 41.5432)
  line L67 (119.9688, 41.5432) -> (119.2103, 41.5432)
  line L68 (119.2103, 41.5432) -> (119.2103, 46.0457)
  line L69 (119.2103, 46.0457) -> (119.9688, 46.0457)
  line L70 (119.9688, 46.0457) -> (119.9688, 45.3747)
  spline S80 degree 2 poles (119.9688, 45.3747) (120.3821, 45.7442) (120.9996, 46.0457) (121.2913, 46.0457) knots 0 0 0 1 2 2 2
  spline S81 degree 2 poles (121.2913, 46.0457) (121.408, 46.0457) (121.5247, 46.0359) (121.5977, 46.0213) knots 0 0 0 1 2 2 2
  line L71 (121.5977, 46.0213) -> (121.5977, 45.2337)
  spline S82 degree 2 poles (123.5474, 41.4557) (122.9299, 41.4557) (122.2346, 42.1607) (122.2346, 42.9241) knots 0 0 0 1 2 2 2
  line L72 (122.2346, 42.9241) -> (122.2346, 45.4184)
  line L73 (122.2346, 45.4184) -> (121.7241, 45.4184)
  line L74 (121.7241, 45.4184) -> (121.7241, 46.0457)
  line L75 (121.7241, 46.0457) -> (122.2346, 46.0457)
  line L76 (122.2346, 46.0457) -> (122.2346, 47.339)
  line L77 (122.2346, 47.339) -> (122.9931, 47.339)
  line L78 (122.9931, 47.339) -> (122.9931, 46.0457)
  line L79 (122.9931, 46.0457) -> (124.3886, 46.0457)
  line L80 (124.3886, 46.0457) -> (124.3886, 45.4184)
  line L81 (124.3886, 45.4184) -> (122.9931, 45.4184)
  line L82 (122.9931, 45.4184) -> (122.9931, 43.2742)
  spline S83 degree 2 poles (122.9931, 43.2742) (122.9931, 42.9338) (123.0174, 42.5594) (123.1001, 42.399) knots 0 0 0 1 2 2 2
  spline S84 degree 2 poles (123.1001, 42.399) (123.1682, 42.258) (123.4745, 42.117) (123.737, 42.117) knots 0 0 0 1 2 2 2
  spline S85 degree 2 poles (123.737, 42.117) (123.9218, 42.117) (124.267, 42.2288) (124.3448, 42.2628) knots 0 0 0 1 2 2 2
  line L83 (124.3448, 42.2628) -> (124.3886, 42.2628)
  line L84 (124.3886, 42.2628) -> (124.3886, 41.5821)
  spline S86 degree 2 poles (124.3886, 41.5821) (124.1746, 41.5238) (123.737, 41.4557) (123.5474, 41.4557) knots 0 0 0 1 2 2 2
  point P0 (152.75, 0)
  point P1 (97.25, 42.3)
  point P2 (97.25, 40.3)
  point P3 (97.25, 40.3)
  dimension "d144" = 2
  dimension "d145" = 0
  constraints: 3 midpoint, 2 other
  measures "d144" distance of point (97.25, 42.3) point (97.25, 40.3)
  measures "d145" horizontal distance of point (97.25, 40.3) point (97.25, 42.3)